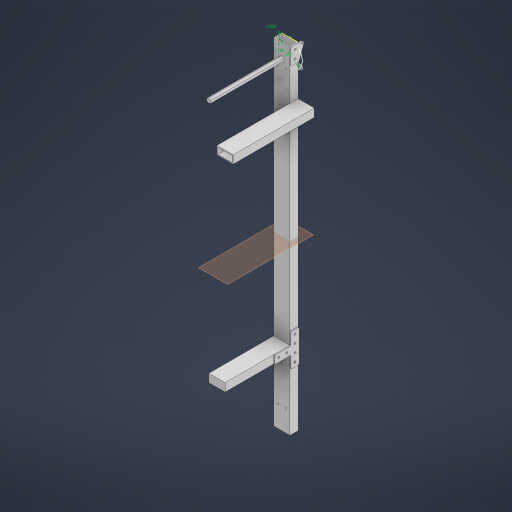
# Autodesk Inventor part: Elevator
Saved by Autodesk Inventor 2023 (Build 270158000, 158)
## iProperties
Created: 2023-01-15
Part Number: Elevator
Material: Generic
Document SubType Name: Modeling
Designer: Terrence
Density: 1 g/cm^3
Appearance: Default
Mass: 822.802 g
Surface Area: 3836.47 cm^2
Volume: 822.802 cm^3
Author: Terrence
Autodesk Inventor part; units mm, degrees
ref_plane "YZ Plane" through (0, 0, 0) normal (1, 0, 0) x (0, 1, 0)
ref_plane "XZ Plane" through (0, 0, 0) normal (0, 1, 0) x (-1, 0, 0)
ref_plane "XY Plane" through (0, 0, 0) normal (0, 0, 1) x (1, 0, 0)
sketch "Sketch1" plane through (0, 0, 0) normal (1, 0, 0) x (0, 1, 0)
  line L0 (1066.8, -361.329) -> (12.7, -361.329)
  line L1 (12.7, -361.329) -> (12.7, -386.729)
  line L2 (12.7, -386.729) -> (1066.8, -386.729)
  line L3 (1066.8, -386.729) -> (1066.8, -361.329)
  point P0 (0, 0)
  dimension "d0" = 1054.1
  dimension "d1" = 25.4
  constraints: 8 end point, 2 parallel, 1 horizontal, 1 perpendicular, 1 vertical
  measures "d0" distance of L2.end L1.end
  measures "d1" distance of L1.end L0.end
extrude "Extrusion1" add sketch "Sketch1" along normal blind 50.8
shell "Shell1" thickness 3.175 removed faces 2 at (16.9333, 1066.8, -378.2623) at (16.9333, 12.7, -369.7956)
sketch "Sketch4" plane through (0, 12.7, -386.729) normal (0, 0, -1) x (-1, 0, 0)
  line L0 (-50.8, 996.95) -> (0, 996.95)
  line L1 (0, 996.95) -> (0, 977.9)
  line L2 (0, 977.9) -> (-50.8, 977.9)
  line L3 (-50.8, 977.9) -> (-50.8, 996.95)
  line L4 (-50.8, 987.425) -> (0, 987.425) construction
  line L5 (-25.4, 996.95) -> (-25.4, 977.9) construction
  circle A0 centre (-57.15, 987.425) radius 3.175
  circle A1 centre (-57.15, 987.425) radius 6.35
  line L6 (-59.5923, 993.2865) -> (-50.8, 996.95)
  line L7 (-59.5923, 981.5635) -> (-50.8, 977.9)
  circle A2 centre (6.35, 987.425) radius 3.175
  circle A3 centre (6.35, 987.425) radius 6.35
  line L8 (8.7923, 993.2865) -> (0, 996.95)
  line L9 (8.7923, 981.5635) -> (0, 977.9)
  line L10 (0, 1054.1) -> (-50.8, 1054.1) projected
  circle A4 centre (-57.15, 987.425) radius 6.35 construction
  dimension "d130" = 50.8
  dimension "d131" = 19.05
  dimension "d132" = 6.35
  dimension "d133" = 12.7
  dimension "d134" = 6.35
  dimension "d185" = 57.15
  dimension "d198" = 12.7
  constraints: 20 end point, 5 centre point, 4 midpoint, 4 point on circle, 4 symmetric about line, 3 coincident, 2 parallel, 2 point on line, 2 tangent, 1 horizontal, 1 perpendicular, 2 other
  measures "d130" distance of L1.end L2.end
  measures "d131" distance of L0.end L1.end
  measures "d132" diameter of A0
  measures "d133" diameter of A1
  measures "d134" distance of L4.start A0.centre
  measures "d185" distance between parallel lines of L10 L0
  measures "d198" diameter of A4
extrude "Extrusion3" add sketch "Sketch4" along normal blind 3.175 separate body
sketch "Sketch5" plane through (0, 12.7, -389.904) normal (0, 0, -1) x (-1, 0, 0)
  line L0 (0, 996.95) -> (-50.8, 996.95) projected
  line L1 (-50.8, 977.9) -> (0, 977.9) projected
  line L2 (0, 996.95) -> (0, 0) projected
  line L3 (0, 996.95) -> (0, 977.9)
  line L4 (0, 987.425) -> (-50.8, 987.425) construction
  line L5 (-50.8, 0) -> (-50.8, 996.95) projected
  circle A0 centre (-12.7, 987.425) radius 2.667
  circle A1 centre (-38.1, 987.425) radius 2.667
  dimension "d135" = 25.4
  dimension "d136" = 12.7
  dimension "d137" = 5.334
  constraints: 4 end point, 3 point on line, 2 centre point, 1 collinear, 1 equal radius, 1 midpoint, 1 perpendicular
  measures "d135" distance of A1.centre A0.centre
  measures "d136" distance of L4.end A1.centre
  measures "d137" diameter of A0
extrude "Extrusion4" cut sketch "Sketch5" against normal through all contours A0 | A1 bodies 2 1
fillet "Fillet1" radius 3.175 4 edges at (50.8, 1009.65, -388.3165) (0, 1009.65, -388.3165) (0, 990.6, -388.3165) (50.8, 990.6, -388.3165)
sketch "Sketch6" plane through (50.8, 0, 0) normal (1, 0, 0) x (0, 0, -1)
  line L0 (361.329, 1066.8) -> (361.329, 12.7) projected
  line L1 (386.729, 12.7) -> (386.729, 1066.8) projected
  line L2 (361.329, 1066.8) -> (386.729, 1066.8)
  line L3 (386.729, 1066.8) -> (386.729, 1016)
  line L4 (386.729, 1016) -> (361.329, 1016)
  line L5 (361.329, 1016) -> (361.329, 1066.8)
  line L6 (386.729, 1066.8) -> (361.329, 1066.8) projected
  arc A0 (402.3167, 1058.8209) -> (398.496, 1065.1673) centre (397.8415, 1060.45) ccw
  circle A1 centre (397.8415, 1060.45) radius 3.175
  circle A2 centre (397.8415, 1060.45) radius 6.35 construction
  line L7 (386.729, 1066.8) -> (398.496, 1065.1673)
  line L8 (402.3167, 1058.8209) -> (386.729, 1016)
  line L9 (386.729, 1066.8) -> (403.0933, 1066.8) construction
  point P0 (0, 0)
  dimension "d33" = 0
  dimension "d34" = 12.7
  dimension "d35" = 9.525
  dimension "d36" = 6.35
  dimension "d37" = 11.1125
  dimension "d225" = 50.8
  dimension "d226" = 6.35
  constraints: 14 end point, 3 centre point, 3 point on line, 3 tangent, 2 coincident, 2 parallel, 2 point on circle, 1 horizontal, 1 perpendicular
  measures "d33" distance between parallel lines of L6 L2
  measures "d34" diameter of A2
  measures "d35" diameter of A0
  measures "d36" diameter of A1
  measures "d37" distance from line of L1 A0.centre
  measures "d225" distance between parallel lines of L2 L4
  measures "d226" vertical distance of L1.end A0.centre
extrude "Extrusion5" add sketch "Sketch6" along normal blind 3.175 separate body
fillet "Fillet2" radius 3.175 3 edges at (52.3875, 1066.8, -361.329) (52.3875, 1016, -361.329) (52.3875, 1016, -386.729)
ref_plane "Work Plane4" through (0, 12.7, -374.029) normal (0, 0, -1) x (-1, 0, 0)
ref_plane "Work Plane8" through (0, 539.75, -361.329) normal (0, 1, 0) x (1, 0, 0)
mirror "Mirror11" about plane through (0, 539.75, -361.329) normal (0, 1, 0) of "Extrusion4" bodies 1
sketch "Sketch16" plane through (0, 12.7, -386.729) normal (0, 0, -1) x (-1, 0, 0)
  circle A0 centre (-25.4, 1009.65) radius 7.3323
  line L0 (-50.165, 977.9) -> (-0.635, 977.9) projected
  line L1 (-25.4, 977.9) -> (-25.4, 939.9108) construction
  circle A1 centre (-25.4, 1009.65) radius 38.1
  line L2 (-25.4, 1016.9823) -> (-19.05, 1013.3162)
  line L3 (-19.05, 1013.3162) -> (-19.05, 1005.9838)
  line L4 (-19.05, 1005.9838) -> (-25.4, 1002.3177)
  line L5 (-25.4, 1002.3177) -> (-31.75, 1005.9838)
  line L6 (-31.75, 1005.9838) -> (-31.75, 1013.3162)
  line L7 (-31.75, 1013.3162) -> (-25.4, 1016.9823)
  line L8 (0, 1054.1) -> (-50.8, 1054.1) projected
  point P0 (0, -12.7)
  point P1 (-25.4, 1054.1)
  dimension "d160" = 76.2
  dimension "d161" = 12.7
  dimension "d186" = 44.45
  constraints: 14 end point, 3 midpoint, 2 coincident, 2 point on line, 1 centre point, 1 vertical, 16 other
  measures "d160" diameter of A1
  measures "d161" distance between parallel lines of L3 L6
  measures "d186" distance of point (-25.4, 1009.65) point (-25.4, 1054.1)
extrude "Extrusion15" cut sketch "Sketch16" against normal through all contours A0 L3 | L2 A0 | L3 L4 L5 L6 L7 L2 | A0 L4 | L7 A0 | A0 L5 | L6 A0 bodies 1
extrude "Extrusion16" add sketch "Sketch16" against normal blind 254 separate body contours L3 L4 L5 L6 L7 L2
sketch "Sketch22" plane through (0, 12.7, -389.904) normal (0, 0, -1) x (-1, 0, 0)
  point P0 (0, -12.7)
sketch "Sketch23" plane through (50.8, 0, 0) normal (1, 0, 0) x (0, 0, -1)
  line L0 (158.129, 257.175) -> (361.329, 257.175)
  line L1 (361.329, 257.175) -> (361.329, 231.775)
  line L2 (361.329, 231.775) -> (158.129, 231.775)
  line L3 (158.129, 231.775) -> (158.129, 257.175)
  line L4 (361.329, 12.7) -> (386.729, 12.7) projected
  point P0 (0, 0)
  dimension "d199" = 203.2
  dimension "d200" = 25.4
  dimension "d201" = 219.075
  constraints: 8 end point, 2 parallel, 1 horizontal, 1 perpendicular, 1 point on line
  measures "d199" distance of L1.end L2.end
  measures "d200" distance of L0.end L1.end
  measures "d201" distance between parallel lines of L4 L2
extrude "Extrusion22" add sketch "Sketch23" against normal up to surface (50.8 mm away) separate body
sketch "Sketch24" plane through (50.8, 0, 0) normal (1, 0, 0) x (0, 0, -1)
  line L0 (361.329, 295.275) -> (386.729, 295.275)
  line L1 (386.729, 295.275) -> (386.729, 193.675)
  line L2 (386.729, 193.675) -> (361.329, 193.675)
  line L3 (361.329, 193.675) -> (361.329, 295.275)
  line L4 (310.529, 257.175) -> (386.729, 257.175)
  line L5 (386.729, 257.175) -> (386.729, 231.775)
  line L6 (386.729, 231.775) -> (310.529, 231.775)
  line L7 (310.529, 231.775) -> (310.529, 257.175)
  line L8 (386.729, 12.7) -> (386.729, 1066.8) projected
  line L9 (361.329, 257.175) -> (158.129, 257.175) projected
  point P0 (0, 0)
  point P1 (386.729, 244.475)
  point P2 (361.329, 257.175)
  point P3 (361.329, 231.775)
  dimension "d204" = 25.4
  dimension "d205" = 25.4
  dimension "d206" = 101.6
  dimension "d207" = 76.2
  constraints: 16 end point, 4 parallel, 3 point on line, 2 horizontal, 2 midpoint, 2 perpendicular
  measures "d204" distance of L6.end L4.start
  measures "d205" distance of L0.start L0.end
  measures "d206" distance of L0.end L1.end
  measures "d207" distance of L5.end L6.end
extrude "Extrusion23" add sketch "Sketch24" along normal blind 3.175 separate body
sketch "Sketch25" plane through (53.975, 0, 0) normal (1, 0, 0) x (0, 0, -1)
  line L0 (386.729, 295.275) -> (361.329, 295.275) projected
  line L1 (374.029, 295.275) -> (374.029, 193.675) construction
  line L2 (361.329, 193.675) -> (386.729, 193.675) projected
  line L3 (310.529, 257.175) -> (310.529, 231.775) projected
  line L4 (310.529, 244.475) -> (386.729, 244.475) construction
  line L5 (386.729, 12.7) -> (386.729, 1066.8) projected
  circle A0 centre (374.029, 282.575) radius 3.175
  point P0 (0, 0)
  dimension "d210" = 6.35
  dimension "d211" = 12.7
  constraints: 4 end point, 4 midpoint, 2 point on line, 1 centre point, 1 perpendicular
  measures "d210" diameter of A0
  measures "d211" distance of point (374.029, 295.275) A0.centre
extrude "Extrusion24" cut sketch "Sketch25" against normal through all bodies 6 1
pattern_linear "Rectangular Pattern6" count 4 spacing 25.4 along (0, -1, 0) of "Extrusion24" bodies 1 6
sketch "Sketch26" plane through (53.975, 0, 0) normal (1, 0, 0) x (0, 0, -1)
  line L0 (310.529, 257.175) -> (310.529, 231.775) projected
  line L1 (310.529, 244.475) -> (386.729, 244.475) construction
  line L2 (386.729, 12.7) -> (386.729, 1066.8) projected
  circle A0 centre (323.229, 244.475) radius 3.175
  line L3 (310.529, 257.175) -> (310.529, 231.775) projected
  point P0 (0, 0)
  dimension "d217" = 6.35
  dimension "d218" = 12.7
  constraints: 2 end point, 2 midpoint, 2 point on line, 1 centre point, 1 horizontal
  measures "d217" diameter of A0
  measures "d218" distance of point (310.529, 244.475) A0.centre
extrude "Extrusion25" cut sketch "Sketch26" against normal through all bodies 6 5
pattern_linear "Rectangular Pattern7" count 2 spacing 25.4 along (0, 0, -1) of "Extrusion25" bodies 6 5
fillet "Fillet13" radius 3.175 8 edges at (52.3875, 295.275, -361.329) (52.3875, 295.275, -386.729) (52.3875, 193.675, -386.729) (52.3875, 193.675, -361.329) (52.3875, 231.775, -310.529) (52.3875, 257.175, -310.529) (52.3875, 231.775, -361.329) (52.3875, 257.175, -361.329)
sketch "Sketch27" plane through (53.975, 0, 0) normal (1, 0, 0) x (0, 0, -1)
  line L0 (374.5049, 1066.8) -> (374.5049, 1016) construction
  line L1 (364.504, 1016) -> (384.5059, 1016) projected
  line L2 (386.729, 1066.8) -> (364.504, 1066.8) projected
  circle A0 centre (374.5049, 1054.1) radius 3.175
  circle A1 centre (374.5049, 1028.7) radius 3.175
  point P0 (0, 0)
  dimension "d227" = 6.35
  dimension "d228" = 6.35
  dimension "d229" = 25.4
  dimension "d230" = 12.7
  constraints: 3 point on line, 2 centre point, 2 end point, 2 midpoint, 1 vertical
  measures "d227" diameter of A0
  measures "d228" diameter of A1
  measures "d229" distance of A1.centre A0.centre
  measures "d230" distance of point (374.505, 1016) A1.centre
extrude "Extrusion26" cut sketch "Sketch27" against normal through all bodies 3 1
sketch "Sketch28" plane through (50.8, 0, 0) normal (1, 0, 0) x (0, 0, -1)
  line L0 (132.729, 913.4701) -> (386.729, 913.4701)
  line L1 (386.729, 913.4701) -> (386.729, 888.0701)
  line L2 (386.729, 888.0701) -> (132.729, 888.0701)
  line L3 (132.729, 888.0701) -> (132.729, 913.4701)
  line L4 (386.729, 12.7) -> (386.729, 1066.8) projected
  arc A0 (364.504, 1066.8) -> (361.329, 1063.625) centre (364.504, 1063.625) ccw projected
  point P0 (0, 0)
  point P1 (362.2589, 1065.8701)
  dimension "d233" = 254
  dimension "d234" = 25.4
  dimension "d235" = 152.4
  constraints: 8 end point, 2 parallel, 1 horizontal, 1 perpendicular, 1 point on circle, 1 point on line
  measures "d233" distance of L1.end L2.end
  measures "d234" distance of L0.end L1.end
  measures "d235" distance from line of point (362.259, 1065.87) L0
extrude "Extrusion27" add sketch "Sketch28" along normal blind 50.8 separate body
shell "Shell4" thickness 3.175 removed faces 2 at (84.6667, 896.5367, -386.729) at (84.6667, 905.0034, -132.729) bodies 7
body "Solid1"
body "Solid3"
body "Solid4"
body "Solid7"
body "Solid9"
body "Solid10"
body "Solid11"
